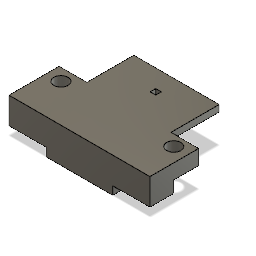
System_Base (Autodesk Fusion 360 archive; units mm, degrees)
design "sensor slit"
Autodesk Fusion 360 part; units mm, degrees
sketch "board contact" plane through (0, 0, 0) normal (0, 1, 0) x (1, 0, 0)
  line L0 (12.7, -1.75) -> (-12.7, -1.75)
  line L1 (-12.7, -1.75) -> (-12.7, 1.75)
  line L2 (-12.7, 1.75) -> (12.7, 1.75)
  line L3 (12.7, 1.75) -> (12.7, -1.75)
  line L4 (61.7395, 0) -> (-97.655, 0) construction
  line L5 (0, -60.5274) -> (0, 48.7233) construction
  line L6 (8.2, 2.75) -> (12.7, 2.75)
  line L7 (12.7, 2.75) -> (12.7, 1.75)
  line L8 (12.7, 1.75) -> (8.2, 1.75)
  line L9 (8.2, 1.75) -> (8.2, 2.75)
  line L10 (-12.7, 3) -> (2.45, 3)
  line L11 (2.45, 3) -> (2.45, 1.75)
  line L12 (2.45, 1.75) -> (-12.7, 1.75)
  line L13 (-12.7, 1.75) -> (-12.7, 3)
  circle A0 centre (10.16, 0.79) radius 1.27
  circle A1 centre (-10.16, 0.79) radius 1.27
  line L14 (-10.16, 0.79) -> (10.16, 0.79) construction
  line L15 (2.45, 9.25) -> (-1.95, 9.25)
  line L16 (-1.95, 9.25) -> (-1.95, 3)
  line L17 (-1.95, 3) -> (2.45, 3)
  line L18 (2.45, 3) -> (2.45, 9.25)
  line L19 (0.5, 7.19) -> (-0.5, 7.19)
  line L20 (-0.5, 7.19) -> (-0.5, 8.19)
  line L21 (-0.5, 8.19) -> (0.5, 8.19)
  line L22 (0.5, 8.19) -> (0.5, 7.19)
  line L23 (7.7, 11.45) -> (-7.7, 11.45)
  line L24 (-7.7, 11.45) -> (-7.7, -1.75)
  line L25 (-7.7, -1.75) -> (7.7, -1.75)
  line L26 (7.7, -1.75) -> (7.7, 11.45)
  line L27 (8.2, 2.75) -> (7.7, 2.75)
  line L28 (-0.5, 7.69) -> (0.5, 7.69) construction
  dimension "d1" = 3.5
  dimension "d2" = 25.4
  dimension "d3" = 4.5
  dimension "d4" = 4.5
  dimension "d7" = 4.75
  dimension "d10" = 20.32
  dimension "d11" = 2.54
  dimension "d12" = 2.54
  dimension "d13" = 10.25
  dimension "d14" = 10.75
  dimension "d15" = 11
  dimension "d17" = 1
  dimension "d18" = 1
  dimension "d20" = 5
  dimension "d21" = 5
  dimension "d22" = 13.2
  dimension "d39" = 9.44
  constraint horizontal L0
  constraint vertical L1
  constraint horizontal L2
  constraint vertical L3
  constraint perpendicular L3 L4
  constraint vertical L5
  constraint coincident origin L5
  constraint coincident origin L4
  constraint symmetric L1 L3 L5
  constraint symmetric L0 L2 L4
  constraint horizontal L6
  constraint vertical L7
  constraint horizontal L8
  constraint vertical L9
  constraint collinear L3 L7
  constraint collinear L2 L8
  constraint horizontal L10
  constraint vertical L11
  constraint horizontal L12
  constraint vertical L13
  constraint collinear L1 L13
  constraint collinear L2 L12
  constraint equal A0 A1
  constraint coincident A1.centre L14.start
  constraint coincident A0.centre L14.end
  constraint horizontal L14
  constraint symmetric L5 A0.centre A1.centre
  constraint horizontal L15
  constraint vertical L16
  constraint horizontal L17
  constraint vertical L18
  constraint collinear L10 L17
  constraint collinear L11 L18
  constraint horizontal L19
  constraint vertical L20
  constraint horizontal L21
  constraint vertical L22
  constraint symmetric L5 L20 L22
  constraint horizontal L23
  constraint vertical L24
  constraint horizontal L25
  constraint vertical L26
  constraint collinear L0 L25
  constraint coincident L26 L27.end
  constraint perpendicular L26 L27
  constraint midpoint L20 L28.start
  constraint midpoint L22 L28.end
  measures "d1" distance of L0.end L1.end
  measures "d2" distance of L0.start L0.end
  measures "d3" distance of L0 L6
  measures "d4" distance of L6.start L6.end
  measures "d7" distance of L0 L10
  measures "d10" distance of A0.centre A1.centre
  measures "d11" distance of L0 A0.centre
  measures "d12" diameter of A0
  measures "d13" distance of L3 L18
  measures "d14" distance of L1 L16
  measures "d15" distance of L0 L15
  measures "d17" distance of L19.start L19.end
  measures "d18" distance of L19.end L20.end
  measures "d20" distance of L3 L26
  measures "d21" distance of L13 L24
  measures "d22" distance of L0 L23
  measures "d39" distance of L0 L28
extrude "Extrude1" add sketch "board contact" along normal blind 3.2 contours L0 L2 L3 L8 A0 L26 | L0 L2 L12 L24 L25 L26 | L2 L6 L7 L8 L9 A0 | L0 L1 L2 L12 A1 L24 | L2 L9 L26 L27 | L2 L10 L11 L15 L16 L18 L23 L24 L26 | L2 L10 L11 L12 L17 L24 | L2 L10 L12 L13 A1 L24 | L10 L15 L16 L17 L18
extrude "Extrude2" cut sketch "board contact" along normal blind 2 contours L2 L9 L26 L27 | L2 L10 L11 L15 L16 L18 L23 L24 L26 | L2 L10 L11 L12 L17 L24 | L10 L15 L16 L17 L18
sketch "vertical extension" plane through (0, 0, 0) normal (0, -1, 0) x (1, 0, 0)
  line L0 (-12.7, -3) -> (-7.7, -3)
  line L1 (-7.7, -1.75) -> (8.2, -1.75)
  line L2 (8.2, -1.75) -> (8.2, -2.75)
  line L3 (8.2, -2.75) -> (12.7, -2.75)
  line L4 (12.7, -2.75) -> (12.7, 1.75)
  line L5 (12.7, 1.75) -> (-12.7, 1.75)
  line L6 (-12.7, 1.75) -> (-12.7, -3)
  circle A0 centre (10.16, -0.79) radius 1.27
  circle A1 centre (-10.16, -0.79) radius 1.27
  line L7 (-6, 6.05) -> (6, 6.05)
  line L8 (6, 6.05) -> (6, 4.55)
  line L9 (6, 4.55) -> (-6, 4.55)
  line L10 (-6, 4.55) -> (-6, 6.05)
  line L11 (0, 1.75) -> (0, -6.45) construction
  line L12 (-12.7, 6.05) -> (12.7, 6.05)
  line L13 (12.7, 6.05) -> (12.7, 1.75)
  line L14 (12.7, 1.75) -> (-12.7, 1.75)
  line L15 (-12.7, 1.75) -> (-12.7, 6.05)
  line L16 (-7.7, -3) -> (-7.7, -1.75)
  dimension "d25" = 12
  dimension "d26" = 1.5
  dimension "d29" = 4.3
  constraint horizontal L7
  constraint vertical L8
  constraint horizontal L9
  constraint vertical L10
  constraint midpoint L5 L11.start
  constraint perpendicular L5 L11
  constraint symmetric L8 L10 L11
  constraint horizontal L12
  constraint vertical L13
  constraint horizontal L14
  constraint vertical L15
  constraint collinear L4 L13
  constraint collinear L6 L15
  constraint collinear L7 L12
  constraint collinear L5 L14
  measures "d25" distance of L7.start L7.end
  measures "d26" distance of L7.end L8.end
  measures "d29" distance of L12.start L5.end
extrude "Extrude4" add sketch "vertical extension" along normal blind -3.2 and the other way blind -1.6 contours L5 L8 L9 L10 L12 L13 L14 L15 | L7 L8 L9 L10 L12
extrude "Extrude3" add sketch "vertical extension" along normal blind 3.1 contours L7 L8 L9 L10 L12
extrude "Extrude6" cut 1 faces at (-2.5667, 0, -0.6331) along direction (0, 1, 0) blind 0.5

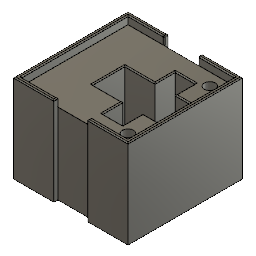
design "button mount v2"
Autodesk Fusion 360 part; units mm, degrees
ref_plane "WorkPlane1" through (0, 0, 12.125) normal (0, 1, 0) x (0, 0, 1)
sketch "face" plane through (0, 0, 12.125) normal (0, 1, 0) x (0, 0, 1)
  line L0 (0, 23) -> (0, -23) construction
  line L1 (-28, 0) -> (21, 0) construction
  line L2 (0, 13.2) -> (-13.2, 13.2)
  line L3 (9, 2.7) -> (4, 2.7)
  line L4 (0, -14.2) -> (0, -13.2)
  line L5 (14.2, -14.2) -> (13.2, -14.2)
  line L6 (13.2, -4.2) -> (14.2, -4.2)
  line L7 (13.2, 13.2) -> (13.2, -13.2)
  line L8 (4, 7.7) -> (4, 13.2)
  line L9 (13.2, -13.2) -> (13.2, -4.2)
  line L10 (-13.2, -13.2) -> (-13.2, -4.2)
  line L11 (0, -13.2) -> (13.2, -13.2)
  line L12 (14.2, -4.2) -> (14.2, -14.2)
  line L13 (12.7, 12.7) -> (12.7, -12.7) construction
  line L14 (9, 7.7) -> (9, 2.7)
  line L15 (-4, 2.7) -> (-4, -4.8)
  line L16 (4, 7.7) -> (9, 7.7)
  line L17 (0, 14.2) -> (0, 13.2)
  line L18 (0, 13.2) -> (13.2, 13.2)
  circle A0 centre (10.16, 10.16) radius 1.375
  line L19 (4, -4.8) -> (4, 2.7)
  line L20 (-13.2, 13.2) -> (13.2, 13.2)
  line L21 (-12.7, -12.7) -> (-12.7, 12.7) construction
  line L22 (-13.2, 13.2) -> (-13.2, 4.2)
  line L23 (14.2, 14.2) -> (13.2, 14.2)
  line L24 (13.2, -13.2) -> (-13.2, -13.2)
  line L25 (13.2, 14.2) -> (0, 14.2)
  line L26 (-9, 2.7) -> (-9, 7.7)
  line L27 (-4, 2.7) -> (-9, 2.7)
  line L28 (13.2, 13.2) -> (13.2, 4.2)
  line L29 (4, 13.2) -> (-4, 13.2)
  line L30 (13.2, -14.2) -> (0, -14.2)
  line L31 (13.2, 4.2) -> (14.2, 4.2)
  line L32 (14.2, 4.2) -> (14.2, 14.2)
  line L33 (-9, 7.7) -> (-4, 7.7)
  line L34 (-14.2, -14.2) -> (-13.2, -14.2)
  line L35 (12.7, -12.7) -> (-12.7, -12.7) construction
  line L36 (-13.2, 4.2) -> (-14.2, 4.2)
  line L37 (-12.7, 0) -> (12.7, 0) construction
  line L38 (-13.2, -14.2) -> (0, -14.2)
  line L39 (-4, -4.8) -> (4, -4.8)
  line L40 (0, -14.2) -> (0, -13.2)
  line L41 (-13.2, -4.2) -> (-14.2, -4.2)
  line L42 (0, 12.7) -> (0, -12.7) construction
  line L43 (0, 14.2) -> (0, 13.2)
  line L44 (-14.2, -4.2) -> (-14.2, -14.2)
  line L45 (-12.7, 12.7) -> (12.7, 12.7) construction
  line L46 (-14.2, 14.2) -> (-13.2, 14.2)
  line L47 (-14.2, 4.2) -> (-14.2, 14.2)
  line L48 (0, -13.2) -> (-13.2, -13.2)
  line L49 (-13.2, 14.2) -> (0, 14.2)
  circle A1 centre (-10.16, 10.16) radius 1.375
  line L50 (-13.2, -13.2) -> (-13.2, 13.2)
  line L51 (-4, 13.2) -> (-4, 7.7)
  circle A2 centre (0, 5.25) radius 4.5 construction
  dimension "d284" = 25.4
  dimension "d285" = 25.4
  dimension "d286" = 2.75
  dimension "d287" = 2.54
  dimension "d288" = 2.54
  dimension "d289" = 2.54
  dimension "d290" = 2.54
  dimension "d291" = 26.4
  dimension "d292" = 26.4
  dimension "d293" = 18
  dimension "d294" = 8
  dimension "d295" = 5
  dimension "d296" = 10.5
  dimension "d297" = 18
  dimension "d298" = 10
  dimension "d299" = 14.2
  dimension "d300" = 1
  dimension "d301" = 1
  dimension "d31" = 17.95
  dimension "d32" = 9
  constraint vertical L0
  constraint horizontal L1
  constraint coincident origin L1
  constraint coincident origin L0
  constraint horizontal L45
  constraint vertical L13
  constraint horizontal L35
  constraint vertical L21
  constraint equal A0 A1
  constraint horizontal L20
  constraint vertical L7
  constraint horizontal L24
  constraint vertical L50
  constraint midpoint L42.start L45
  constraint midpoint L42.end L35
  constraint midpoint L37.start L21
  constraint midpoint L37.end L13
  constraint symmetric L7 L42 L50
  constraint symmetric L20 L24 L37
  constraint horizontal L39
  constraint vertical L19
  constraint horizontal L29
  constraint vertical L51
  constraint collinear L20 L29
  constraint horizontal L33
  constraint vertical L14
  constraint horizontal L3
  constraint vertical L26
  constraint coincident L15.start L3
  constraint collinear L15 L51
  constraint collinear L16 L33
  constraint collinear L3 L27
  constraint collinear L8 L19
  constraint horizontal L46
  constraint vertical L22
  constraint horizontal L36
  constraint vertical L47
  constraint horizontal L49
  constraint vertical L43
  constraint horizontal L2
  constraint collinear L2 L20
  constraint collinear L22 L50
  constraint symmetric L46.start L23.start L42
  constraint symmetric L46.end L23.end L42
  constraint symmetric L28.end L22.end L42
  constraint symmetric L31.end L36.end L42
  constraint symmetric L17.start L25.end L42
  constraint symmetric L2.start L17.end L42
  constraint symmetric L2.end L7.start L42
  constraint symmetric L34.start L46.start L37
  constraint symmetric L34.end L46.end L37
  constraint symmetric L10.end L22.end L37
  constraint symmetric L36.end L41.end L37
  constraint symmetric L17.start L4.start L37
  constraint symmetric L2.start L4.end L37
  constraint symmetric L10.start L2.end L37
  constraint symmetric L28.end L6.start L37
  constraint symmetric L31.end L6.end L37
  constraint symmetric L23.start L5.start L37
  constraint symmetric L23.end L5.end L37
  constraint symmetric L7.start L7.end L37
  constraint collinear L0 L42
  constraint collinear L1 L37
  constraint coincident L42 A2.centre
  measures "d284" distance of L13.start L21.end
  measures "d285" distance of L13.start L13.end
  measures "d286" diameter of A1
  measures "d287" distance of A1.centre L45
  measures "d288" distance of A1.centre L21
  measures "d289" distance of A0.centre L45
  measures "d290" distance of A0.centre L13
  measures "d291" distance of L7.start L2.end
  measures "d292" distance of L7.end L7.start
  measures "d293" distance of L19.start L8.end
  measures "d294" distance of L19.start L15.end
  measures "d295" distance of L14.start L3.start
  measures "d296" distance of L3 L20
  measures "d297" distance of L3.start L26.start
  measures "d298" distance of L46.start L36.end
  measures "d299" distance of L43 L47
  measures "d300" distance of L17.start L2.start
  measures "d301" distance of L36.end L22.end
  measures "d31" distance of L35 A2.centre
  measures "d32" diameter of A2
ref_plane "WorkPlane2" through (0, -20, 0) normal (0, 1, 0) x (0, 0, 1)
extrude "Extrude1" add sketch "face" against normal up to surface (20 mm away) contours L2 L3 L7 L8 L9 L10 L11 L14 L15 L16 L18 L19 L20 L22 L24 L26 L27 L28 L33 L39 L48 L50 L51 | A0 | A1
extrude "Extrude3" cut sketch "face" against normal blind 13 contours A0 | A1
extrude "Extrude4" add sketch "face" along normal blind 2 and the other way up to surface (20 mm away) contours L2 L17 L20 L22 L29 L36 L43 L46 L47 L49 L50 | L7 L17 L18 L20 L23 L25 L28 L29 L31 L32 L43 | L4 L10 L24 L34 L38 L40 L41 L44 L48 L50 | L4 L5 L6 L7 L9 L11 L12 L24 L30 L40
fillet "Fillet3" radius 0.25 8 edges at (8.7, 2, -1.075) (4.2, 1, -1.075) (-4.2, 1, -1.075) (-8.7, 2, -1.075) (-13.2, 2, 12.125) (13.2, 2, 12.125) (-8.7, 2, 25.325) (8.7, 2, 25.325)
fillet "Fillet3" radius 0.25 11 edges at (10.45, 0, 8.125) (7.7, 0, 5.625) (5.2, 0, 3.125) (2.7, 0, 5.625) (-1.05, 0, 8.125) (-4.8, 0, 12.125) (-1.05, 0, 16.125) (2.7, 0, 18.625) (5.2, 0, 21.125) (7.7, 0, 18.625) (10.45, 0, 16.125)
fillet "Fillet3" radius 0.25 10 edges at (9.2, 2, -2.075) (4.2, 2, -1.575) (-4.2, 2, -1.575) (-9.2, 2, -2.075) (-14.2, 2, 12.125) (-9.2, 2, 26.325) (-4.2, 2, 25.825) (4.2, 2, 25.825) (9.2, 2, 26.325) (14.2, 2, 12.125)
equation "FACE_DEG = 0 deg"
equation "d289 = d263"
equation "d290 = d264"
equation "d291 = 26.10 mm + 2 * 0.15 mm"
equation "d292 = 26.10 mm + 2 * 0.15 mm"
equation "HEIGHT = -20 mm"

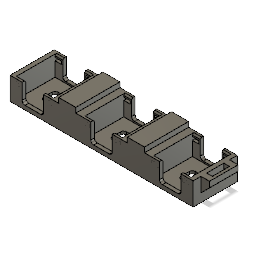
design "magnet storage v4"
Autodesk Fusion 360 part; units mm, degrees
sketch "base" plane through (0, 0, 0) normal (0, 1, 0) x (1, 0, 0)
  line L0 (-64, 15.5) -> (64, 15.5)
  line L1 (64, 15.5) -> (64, -15.5)
  line L2 (64, -15.5) -> (-64, -15.5)
  line L3 (-64, -15.5) -> (-64, 15.5)
  line L4 (64, 0) -> (-64, 0) construction
  line L5 (0, 15.5) -> (0, -15.5) construction
  line L6 (-61, 13) -> (-35, 13)
  line L7 (-35, 13) -> (-35, -13)
  line L8 (-35, -13) -> (-61, -13)
  line L9 (-61, -13) -> (-61, 13)
  line L10 (-53, 5) -> (-43, 5)
  line L11 (-43, 5) -> (-43, -5)
  line L12 (-43, -5) -> (-53, -5)
  line L13 (-53, -5) -> (-53, 5)
  line L14 (-48, 13) -> (-48, -13) construction
  line L15 (-13, 13) -> (13, 13)
  line L16 (-13, -13) -> (-13, 13)
  line L17 (13, -13) -> (-13, -13)
  line L18 (5, -5) -> (-5, -5)
  line L19 (-5, -5) -> (-5, 5)
  line L20 (-5, 5) -> (5, 5)
  line L21 (5, 5) -> (5, -5)
  line L22 (13, 13) -> (13, -13)
  line L23 (35, 13) -> (61, 13)
  line L24 (35, -13) -> (35, 13)
  line L25 (61, -13) -> (35, -13)
  line L26 (53, -5) -> (43, -5)
  line L27 (43, -5) -> (43, 5)
  line L28 (43, 5) -> (53, 5)
  line L29 (53, 5) -> (53, -5)
  line L30 (61, 13) -> (61, -13)
  dimension "d2" = 31
  dimension "d3" = 26
  dimension "d4" = 10
  dimension "d5" = 3
  dimension "d8" = 48
  dimension "d9" = 0
  dimension "d86" = 3
  constraint horizontal L0
  constraint vertical L1
  constraint horizontal L2
  constraint vertical L3
  constraint midpoint L1 L4.start
  constraint midpoint L3 L4.end
  constraint midpoint L0 L5.start
  constraint midpoint L2 L5.end
  constraint coincident origin L5
  constraint coincident origin L4
  constraint horizontal L6
  constraint vertical L7
  constraint horizontal L8
  constraint vertical L9
  constraint horizontal L10
  constraint vertical L11
  constraint horizontal L12
  constraint vertical L13
  constraint equal L6 L7
  constraint equal L10 L11
  constraint symmetric L4 L6 L8
  constraint midpoint L6 L14.start
  constraint midpoint L8 L14.end
  constraint symmetric L4 L10 L12
  constraint symmetric L11 L13 L14
  measures "d2" distance of L0.start L2.end
  measures "d3" distance of L6.start L8.end
  measures "d4" distance of L10.start L10.end
  measures "d5" distance of L3 L9
  measures "d86" distance of L1 L30
extrude "Extrude1" add sketch "base" along normal blind 2 contours L6 L7 L8 L9 | L15 L16 L17 L22 | L23 L24 L25 L30 makes body 1 at (10.3333, 0, -1.6667) makes body 2 at (58.3333, 0, 1.6667) makes body 3 at (-58.3333, 0, 1.6667)
extrude "Extrude2" add sketch "base" along normal blind 12 contours L0 L1 L2 L3 bodies 1 2 3
sketch "access slots" plane through (0, 0, 15.5) normal (0, 0, 1) x (1, 0, 0)
  line L0 (-64, 0) -> (64, 0)
  line L1 (64, 0) -> (64, 12)
  line L2 (64, 12) -> (-64, 12)
  line L3 (-64, 12) -> (-64, 0)
  line L4 (-42.5, 3) -> (-53.5, 3)
  line L5 (-55.5, 5) -> (-55.5, 12)
  line L6 (-55.5, 12) -> (-40.5, 12)
  line L7 (-40.5, 12) -> (-40.5, 5)
  line L8 (64, 0) -> (-64, 0)
  line L9 (-48, 12) -> (-48, 3) construction
  arc A0 (-55.5, 5) -> (-53.5, 3) centre (-53.5, 5) ccw
  arc A1 (-42.5, 3) -> (-40.5, 5) centre (-42.5, 5) ccw
  line L10 (-7.5, 5) -> (-7.5, 12)
  line L11 (-7.5, 12) -> (7.5, 12)
  arc A2 (-7.5, 5) -> (-5.5, 3) centre (-5.5, 5) ccw
  line L12 (5.5, 3) -> (-5.5, 3)
  arc A3 (5.5, 3) -> (7.5, 5) centre (5.5, 5) ccw
  line L13 (7.5, 12) -> (7.5, 5)
  line L14 (40.5, 5) -> (40.5, 12)
  line L15 (40.5, 12) -> (55.5, 12)
  arc A4 (40.5, 5) -> (42.5, 3) centre (42.5, 5) ccw
  line L16 (53.5, 3) -> (42.5, 3)
  arc A5 (53.5, 3) -> (55.5, 5) centre (53.5, 5) ccw
  line L17 (55.5, 12) -> (55.5, 5)
  point P0 (-61, 12)
  point P1 (-13, 12)
  point P2 (35, 12)
  point P3 (35, 15)
  dimension "d20" = 3
  dimension "d21" = 15
  dimension "d22" = 13
  dimension "d23" = 2
  dimension "d26" = 48
  dimension "d27" = 0
  constraint horizontal L4
  constraint vertical L5
  constraint horizontal L6
  constraint vertical L7
  constraint midpoint L6 L9.start
  constraint collinear L2 L6
  constraint coincident L4 L9.end
  constraint tangent L4 A0
  constraint tangent L5 A0
  constraint tangent L4 A1
  constraint tangent L7 A1
  constraint equal A0 A1
  constraint midpoint L4 L9.end
  measures "d20" distance of L4 L8
  measures "d21" distance of L5.end L6.end
  measures "d22" distance of P0 L9
  measures "d23" radius of A0
extrude "Extrude3" cut sketch "access slots" against normal up to surface (31 mm away) contours L2 L4 L5 L6 L7 A0 A1 | L2 L14 L15 A4 L16 A5 L17 | L2 L10 L11 A2 L12 A3 L13 bodies 1
fillet "Fillet1" radius 2 12 edges at (-43, 1, 5) (-53, 1, 5) (-53, 1, -5) (-43, 1, -5) (5, 1, -5) (5, 1, 5) (-5, 1, 5) (-5, 1, -5) (43, 1, -5) (43, 1, 5) (53, 1, -5) (53, 1, 5) on bodies 1
ref_plane "WorkPlane1" through (0, 12, 0) normal (0, 1, 0) x (0, 0, 1)
sketch "cover indents" plane through (-24, 12, 0) normal (0, 1, 0) x (1, 0, 0)
  circle A0 centre (-5, 9.5) radius 1.4
  circle A1 centre (-5, 9.5) radius 3
  line L0 (16.5, 15.5) -> (-16.5, 15.5)
  line L1 (-5, 12.5) -> (-11, 12.5)
  line L2 (11, -13) -> (-11, -13)
  circle A2 centre (5, 9.5) radius 1.4
  circle A3 centre (5, 9.5) radius 3
  line L3 (-5, 9.5) -> (5, 9.5) construction
  line L4 (5, 12.5) -> (11, 12.5)
  line L5 (-11, 13) -> (-11, -13)
  line L6 (11, -13) -> (11, 13)
  line L7 (-11, -13) -> (-16.5, -13)
  line L8 (-2, 9.5) -> (-2, 8)
  line L9 (2, 9.5) -> (2, 8)
  circle A4 centre (43, -9.5) radius 1.4
  circle A5 centre (43, -9.5) radius 3
  line L10 (37, 13) -> (37, -13)
  line L11 (31.5, -15.5) -> (64.5, -15.5)
  circle A6 centre (53, -9.5) radius 1.4
  circle A7 centre (53, -9.5) radius 3
  line L12 (43, -9.5) -> (53, -9.5) construction
  line L13 (59, -13) -> (59, 13) construction
  line L14 (43, -12.5) -> (37, -12.5)
  line L15 (59, -12.5) -> (53, -12.5)
  line L16 (37, 13) -> (59, 13)
  line L17 (37, 13) -> (37, -12.5)
  line L18 (59, -13) -> (59, 13)
  line L19 (46, -9.5) -> (46, -6.5)
  line L20 (46, -6.5) -> (50, -6.5)
  line L21 (50, -6.5) -> (50, -9.5)
  line L22 (-2, 8) -> (2, 8)
  dimension "d33" = 2.8
  dimension "d34" = 6
  dimension "d35" = 6
  dimension "d37" = 6
  dimension "d38" = 6
  dimension "d57" = 6
  dimension "d58" = 6
  dimension "d59" = 6
  dimension "d84" = 1.5
  constraint concentric A0 A1
  constraint coincident A1 L1.start
  constraint horizontal L1
  constraint equal A0 A2
  constraint concentric A2 A3
  constraint equal A1 A3
  constraint coincident A0.centre A1.centre
  constraint coincident A2.centre A3.centre
  constraint horizontal L3
  constraint coincident A3 L4.start
  constraint horizontal L4
  constraint coincident L4.end L6
  constraint coincident L1.end L5
  constraint tangent A1 L1
  constraint tangent A3 L4
  constraint coincident L2.end L5
  constraint coincident L2.start L6
  constraint collinear L2 L7
  constraint coincident A1 L8.start
  constraint coincident L3 L8.start
  constraint tangent A1 L8
  constraint coincident A3 L9.start
  constraint coincident L3 L9.start
  constraint tangent A3 L9
  constraint equal A2 A4
  constraint concentric A4 A5
  constraint equal A3 A5
  constraint concentric A6 A7
  constraint equal A4 A6
  constraint equal A5 A7
  constraint coincident A4.centre A5.centre
  constraint coincident A6.centre A7.centre
  constraint horizontal L12
  constraint coincident A5 L14.start
  constraint coincident L10 L14.end
  constraint tangent A5 L14
  constraint horizontal L14
  constraint coincident L13 L15.start
  constraint coincident A7 L15.end
  constraint perpendicular L13 L15
  constraint tangent A7 L15
  constraint coincident L10.start L16.start
  constraint coincident L13.end L16.end
  constraint coincident L13.start L18.start
  constraint coincident A5 L19.start
  constraint coincident L12 L19.start
  constraint tangent A5 L19
  constraint perpendicular L18 L20
  constraint coincident A7 L21.end
  constraint coincident L12 L21.end
  constraint tangent A7 L21
  constraint tangent A5 L20
  constraint equal L8 L9
  measures "d33" diameter of A0
  measures "d34" diameter of A1
  measures "d35" distance of A0.centre L0
  measures "d37" distance of A0.centre L5
  measures "d38" distance of A2.centre L6
  measures "d57" distance of A4.centre L10
  measures "d58" distance of A4.centre L11
  measures "d59" distance of A6.centre L13
  measures "d84" distance of L9.start L9.end
extrude "Extrude9" add 2 faces at (-63, 12, -4.3333) (63, 12, 4.3333) along direction (0, 1, 0) blind 4 on bodies 1 bodies 1
sketch "left top" plane through (0, 12, 0) normal (0, 1, 0) x (-1, 0, 0)
  line L0 (-7.5, -15.5) -> (-7.5, -13)
  line L1 (-7.5, -13) -> (-13, -13)
  line L2 (-13, -13) -> (-13, 13)
  line L3 (-13, 13) -> (-7.5, 13)
  line L4 (-7.5, 13) -> (-7.5, 15.5)
  line L5 (-7.5, 15.5) -> (-40.5, 15.5)
  line L6 (-40.5, 15.5) -> (-40.5, 13)
  line L7 (-40.5, 13) -> (-35, 13)
  line L8 (-35, 13) -> (-35, -13)
  line L9 (-35, -13) -> (-40.5, -13)
  line L10 (-40.5, -13) -> (-40.5, -15.5)
  line L11 (-40.5, -15.5) -> (-7.5, -15.5)
  line L12 (-30, 15.5) -> (-30, -15.5)
  line L13 (-18, 15.5) -> (-18, -15.5)
  dimension "d94" = 5
  dimension "d95" = 5
  dimension "d138" = 12
  constraint coincident L5 L12.start
  constraint coincident L11 L12.end
  constraint perpendicular L11 L12
  constraint coincident L5 L13.start
  constraint coincident L11 L13.end
  constraint perpendicular L11 L13
  measures "d94" distance of L8 L12
  measures "d95" distance of L2 L13
  measures "d138" distance of L12 L13
extrude "Extrude11" add sketch "left top" along normal blind 4 contours L5 L6 L7 L8 L9 L10 L11 L12 bodies 1
ref_plane "WorkPlane4" through (48, 9, 13) normal (0, 0, -1) x (-1, 0, 0)
sketch "left prong holes" plane through (37.75, 13.75, 13) normal (0, 0, -1) x (1, 0, 0)
  line L0 (1.75, -0.25) -> (-2.75, -0.25)
  line L1 (-2.75, -0.25) -> (-2.75, 2)
  line L2 (-2.75, 2) -> (1.75, 2)
  line L3 (1.75, 2) -> (1.75, -0.25)
  line L4 (2.75, -2.25) -> (2.75, 8.75)
  line L5 (18.75, -0.25) -> (23.25, -0.25)
  line L6 (23.25, -0.25) -> (23.25, 2)
  line L7 (23.25, 2) -> (18.75, 2)
  line L8 (18.75, 2) -> (18.75, -0.25)
  line L9 (17.75, 8.75) -> (17.75, -2.25)
  line L10 (-7.75, -2.25) -> (2.75, -2.25)
  line L11 (17.75, -2.25) -> (26.25, -2.25)
  dimension "d119" = 1
  dimension "d120" = 4.5
  dimension "d121" = 2.25
  dimension "d123" = 1
  dimension "d125" = 2.25
  dimension "d132" = 2
  dimension "d133" = 2
  constraint horizontal L0
  constraint vertical L1
  constraint horizontal L2
  constraint vertical L3
  constraint horizontal L5
  constraint vertical L6
  constraint horizontal L7
  constraint vertical L8
  constraint equal L0 L5
  measures "d119" distance of L3 L4
  measures "d120" distance of L0.start L0.end
  measures "d121" distance of L0.end L1.end
  measures "d123" distance of L8 L9
  measures "d125" distance of L5.start L7.end
  measures "d132" distance of L0 L10
  measures "d133" distance of L5 L11
extrude "Extrude16" cut sketch "left prong holes" against normal blind 2 bodies 1
mirror "Mirror1" about plane through (0, 0, 0) normal (0, 0, 1) of "Extrude16"
sketch "right top" plane through (0, 12, 0) normal (0, 1, 0) x (-1, 0, 0)
  line L0 (40.5, -15.5) -> (40.5, -13)
  line L1 (40.5, -13) -> (35, -13)
  line L2 (35, -13) -> (35, 13)
  line L3 (35, 13) -> (40.5, 13)
  line L4 (40.5, 13) -> (40.5, 15.5)
  line L5 (40.5, 15.5) -> (7.5, 15.5)
  line L6 (7.5, 15.5) -> (7.5, 13)
  line L7 (7.5, 13) -> (13, 13)
  line L8 (13, 13) -> (13, -13)
  line L9 (13, -13) -> (7.5, -13)
  line L10 (7.5, -13) -> (7.5, -15.5)
  line L11 (7.5, -15.5) -> (40.5, -15.5)
  line L12 (18, 15.5) -> (18, -15.5)
  line L13 (30, 15.5) -> (30, -15.5)
  dimension "d141" = 5
  dimension "d142" = 5
  constraint coincident L5 L12.start
  constraint coincident L11 L12.end
  constraint perpendicular L11 L12
  constraint coincident L5 L13.start
  constraint coincident L11 L13.end
  constraint perpendicular L11 L13
  measures "d141" distance of L8 L12
  measures "d142" distance of L2 L13
extrude "Extrude17" add sketch "right top" sketch "left top" along normal blind 7.5 contours L5 L11 L12 L13 of sketch 2 contours L5 L11 L12 L13 bodies 1
extrude "Extrude18" add sketch "left top" 2 faces at (-16.3333, 12, -4.3333) (-31.6667, 12, 4.3333) along normal blind 4 contours L0 L1 L2 L3 L4 L5 L11 L13 on bodies 1 bodies 1
sketch "middle prong holes" plane through (0, 0, 13) normal (0, 0, -1) x (-1, 0, 0)
  line L0 (-7.5, 5) -> (-7.5, 16)
  line L1 (-7.5, 16) -> (-13, 16)
  line L2 (-13, 16) -> (-13, 2)
  line L3 (-13, 2) -> (13, 2)
  line L4 (13, 2) -> (13, 16)
  line L5 (13, 16) -> (7.5, 16)
  line L6 (7.5, 16) -> (7.5, 5)
  arc A0 (5.5, 3) -> (7.5, 5) centre (5.5, 5) ccw
  line L7 (5.5, 3) -> (-5.5, 3)
  arc A1 (-7.5, 5) -> (-5.5, 3) centre (-5.5, 5) ccw
  line L8 (-13, 14) -> (-8.5, 14)
  line L9 (-8.5, 14) -> (-8.5, 12)
  line L10 (-8.5, 12) -> (-13, 12)
  line L11 (-13, 12) -> (-13, 14)
  line L12 (8.5, 14) -> (13, 14)
  line L13 (13, 14) -> (13, 12)
  line L14 (13, 12) -> (8.5, 12)
  line L15 (8.5, 12) -> (8.5, 14)
  dimension "d145" = 2
  dimension "d146" = 1
  dimension "d147" = 4.5
  dimension "d148" = 2
  dimension "d149" = 1
  constraint horizontal L8
  constraint vertical L9
  constraint horizontal L10
  constraint vertical L11
  constraint horizontal L12
  constraint vertical L13
  constraint horizontal L14
  constraint vertical L15
  constraint collinear L8 L12
  constraint collinear L10 L14
  constraint equal L8 L12
  measures "d145" distance of L1 L8
  measures "d146" distance of L0 L9
  measures "d147" distance of L8.start L8.end
  measures "d148" distance of L8.end L9.end
  measures "d149" distance of L6 L15
sketch "right prong holes" plane through (0, 0, 13) normal (0, 0, -1) x (-1, 0, 0)
  line L0 (40.5, 5) -> (40.5, 16)
  line L1 (40.5, 16) -> (35, 16)
  line L2 (35, 16) -> (35, 2)
  line L3 (35, 2) -> (61, 2)
  line L4 (61, 2) -> (61, 16)
  line L5 (61, 16) -> (55.5, 16)
  line L6 (55.5, 16) -> (55.5, 5)
  arc A0 (53.5, 3) -> (55.5, 5) centre (53.5, 5) ccw
  line L7 (53.5, 3) -> (42.5, 3)
  arc A1 (40.5, 5) -> (42.5, 3) centre (42.5, 5) ccw
  line L8 (35, 14) -> (39.5, 14)
  line L9 (39.5, 14) -> (39.5, 12)
  line L10 (39.5, 12) -> (35, 12)
  line L11 (35, 12) -> (35, 14)
  line L12 (56.5, 14) -> (61, 14)
  line L13 (61, 14) -> (61, 12)
  line L14 (61, 12) -> (56.5, 12)
  line L15 (56.5, 12) -> (56.5, 14)
  dimension "d150" = 1
  dimension "d151" = 2
  dimension "d152" = 4.5
  dimension "d153" = 2
  dimension "d154" = 1
  constraint horizontal L8
  constraint vertical L9
  constraint horizontal L10
  constraint vertical L11
  constraint horizontal L12
  constraint vertical L13
  constraint horizontal L14
  constraint vertical L15
  constraint equal L8 L12
  constraint collinear L8 L12
  constraint collinear L10 L14
  measures "d150" distance of L0 L9
  measures "d151" distance of L1 L8
  measures "d152" distance of L8.start L8.end
  measures "d153" distance of L8.end L9.end
  measures "d154" distance of L6 L15
extrude "Extrude19" cut sketch "middle prong holes" sketch "right prong holes" along normal blind 28 and the other way blind 2 contours L2 L8 L9 L10 L11 | L4 L12 L13 L14 L15 of sketch 2 contours L2 L8 L9 L10 L11 | L4 L12 L13 L14 L15 bodies 1
chamfer "Chamfer2" distance 1 angle 45 2 edges at (37.75, 16, 13) (58.25, 16, 13) on bodies 1
chamfer "Chamfer2" distance 1 angle 45 2 edges at (37.75, 16, -13) (58.25, 16, -13) on bodies 1
chamfer "Chamfer2" distance 1 angle 45 8 edges at (10.25, 16, 13) (-10.25, 16, 13) (10.25, 16, -13) (-10.25, 16, -13) (-37.75, 16, 13) (-58.25, 16, 13) (-58.25, 16, -13) (-37.75, 16, -13) on bodies 1
sketch "handle" plane through (64, 0, 0) normal (1, 0, 0) x (0, 0, -1)
  line L0 (-15.5, 0) -> (15.5, 0)
  line L1 (15.5, 0) -> (15.5, 16)
  line L2 (-15.5, 16) -> (-15.5, 0)
  line L3 (-10, 16) -> (10, 16)
  line L4 (10, 16) -> (10, 12)
  line L5 (10, 12) -> (-10, 12)
  line L6 (-10, 12) -> (-10, 16)
  line L7 (0, 19) -> (0, 0) construction
  line L8 (-6, 16) -> (-6, 12)
  line L9 (6, 16) -> (6, 12)
  line L10 (15.5, 16) -> (-15.5, 16)
  dimension "d73" = 20
  dimension "d74" = 4
  dimension "d76" = 4
  dimension "d77" = 4
  constraint horizontal L3
  constraint vertical L4
  constraint horizontal L5
  constraint vertical L6
  constraint coincident L7.end origin
  constraint symmetric L4 L6 L7
  constraint coincident L3 L8.start
  constraint coincident L5 L8.end
  constraint perpendicular L5 L8
  constraint coincident L3 L9.start
  constraint coincident L5 L9.end
  constraint perpendicular L5 L9
  measures "d73" distance of L3.start L3.end
  measures "d74" distance of L3.start L5.end
  measures "d76" distance of L4 L9
  measures "d77" distance of L6 L8
extrude "Extrude7" add sketch "handle" along normal blind 6 contours L3 L5 L6 L8 L10 | L3 L4 L5 L9 L10 | L3 L5 L8 L9 L10 bodies 1
extrude "Extrude8" cut sketch "handle" along normal blind 4 contours L3 L5 L8 L9 L10 bodies 1
draft "Draft1" angle 45 neutral plane through (70, 0, 0) pull (1, 0, 0) 1 faces at (67.3333, 12, -8.6667) on bodies 1
equation "d38 = d37"
equation "d57 = d37"
equation "d58 = d35"
equation "d59 = d37"
equation "d77 = d76"
equation "d95 = d94"
equation "d123 = d119"
equation "d142 = d141"
equation "d149 = d146"
equation "d154 = d150"

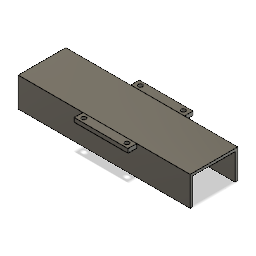
design "magnet storage cover"
Autodesk Fusion 360 part; units mm, degrees
sketch "base" plane through (0, 0, 0) normal (0, 1, 0) x (1, 0, 0)
  line L0 (-67, 15.5) -> (67, 15.5) construction
  line L1 (67, 15.5) -> (67, -15.5) construction
  line L2 (67, -15.5) -> (-67, -15.5) construction
  line L3 (-67, -15.5) -> (-67, 15.5) construction
  line L4 (0, 15.5) -> (0, -15.5) construction
  line L5 (-67, 0) -> (67, 0) construction
  line L6 (-69.25, 17.75) -> (58.75, 17.75)
  line L7 (58.75, 17.75) -> (58.75, 15.75)
  line L8 (58.75, 15.75) -> (-69.25, 15.75)
  line L9 (-69.25, 15.75) -> (-69.25, 17.75)
  line L10 (-69.25, -15.75) -> (58.75, -15.75)
  line L11 (58.75, -15.75) -> (58.75, -17.75)
  line L12 (58.75, -17.75) -> (-69.25, -17.75)
  line L13 (-69.25, -17.75) -> (-69.25, -15.75)
  line L14 (-69.25, 15.75) -> (-69.25, -15.75)
  line L15 (-67.25, -15.75) -> (-67.25, 15.75)
  dimension "d1" = 134
  dimension "d2" = 31
  dimension "d3" = 128
  dimension "d4" = 2
  dimension "d5" = 2
  dimension "margin" = 0.25
  dimension "d7" = 0.25
  dimension "d8" = 0.25
  constraint horizontal L0
  constraint vertical L1
  constraint horizontal L2
  constraint vertical L3
  constraint midpoint L0 L4.start
  constraint midpoint L2 L4.end
  constraint midpoint L3 L5.start
  constraint midpoint L1 L5.end
  constraint coincident origin L5
  constraint coincident origin L4
  constraint horizontal L6
  constraint vertical L7
  constraint horizontal L8
  constraint vertical L9
  constraint horizontal L10
  constraint vertical L11
  constraint horizontal L12
  constraint vertical L13
  constraint collinear L7 L11
  constraint collinear L9 L13
  constraint coincident L10 L15.start
  constraint coincident L8 L15.end
  constraint perpendicular L8 L15
  constraint equal L9 L13
  measures "d1" distance of L0.start L0.end
  measures "d2" distance of L0.start L2.end
  measures "d3" distance of L6.start L6.end
  measures "d4" distance of L6.start L8.end
  measures "d5" distance of L14 L15
  measures "margin" distance of L3 L15
  measures "d7" distance of L2 L10
  measures "d8" distance of L0 L8
extrude "Extrude1" add sketch "base" along normal blind 20 makes body 1
sketch "top" plane through (0, 20, 0) normal (0, 1, 0) x (-1, 0, 0)
  line L0 (-58.75, 15.75) -> (67.25, 15.75)
  line L1 (67.25, 15.75) -> (67.25, -15.75)
  line L2 (67.25, -15.75) -> (-58.75, -15.75)
  line L3 (-58.75, -15.75) -> (-58.75, -17.75)
  line L4 (-58.75, -17.75) -> (69.25, -17.75)
  line L5 (69.25, -17.75) -> (69.25, 17.75)
  line L6 (69.25, 17.75) -> (-58.75, 17.75)
  line L7 (-58.75, 17.75) -> (-58.75, 15.75)
  line L8 (69.25, -17.75) -> (-58.75, -17.75)
  line L9 (-58.75, -17.75) -> (-58.75, 17.75)
  line L10 (-58.75, 17.75) -> (69.25, 17.75)
  line L11 (69.25, 17.75) -> (69.25, -17.75)
  constraint horizontal L8
  constraint vertical L9
  constraint horizontal L10
  constraint vertical L11
  constraint collinear L3 L9
  constraint collinear L5 L11
  constraint collinear L4 L8
  constraint collinear L6 L10
extrude "Extrude2" add sketch "top" along normal blind 2 bodies 1
sketch "wing supports" plane through (0, 22, 0) normal (0, 1, 0) x (-1, 0, 0)
  line L0 (69.25, 17.75) -> (-58.75, 17.75)
  line L1 (-58.75, 17.75) -> (-58.75, -17.75)
  line L2 (-58.75, -17.75) -> (69.25, -17.75)
  line L3 (69.25, -17.75) -> (69.25, 17.75)
  line L4 (21, -24.25) -> (-19, -24.25)
  line L5 (-19, -24.25) -> (-19, -17.75)
  line L6 (-19, -17.75) -> (21, -17.75)
  line L7 (21, -17.75) -> (21, -24.25)
  line L8 (21, 17.75) -> (-19, 17.75)
  line L9 (-19, 17.75) -> (-19, 24.25)
  line L10 (-19, 24.25) -> (21, 24.25)
  line L11 (21, 24.25) -> (21, 17.75)
  circle A0 centre (17, 21) radius 1.55
  circle A1 centre (-15, 21) radius 1.55
  line L12 (17, 21) -> (-15, 21) construction
  circle A2 centre (17, -21) radius 1.55
  circle A3 centre (-15, -21) radius 1.55
  line L13 (17, -21) -> (-15, -21) construction
  circle A4 centre (17, 21) radius 2.75
  circle A5 centre (-15, 21) radius 2.75
  circle A6 centre (17, -21) radius 2.75
  circle A7 centre (-15, -21) radius 2.75
  dimension "d13" = 6.5
  dimension "d14" = 40
  dimension "d15" = 19
  dimension "d16" = 3.1
  dimension "d17" = 3.25
  dimension "d18" = 4
  dimension "d19" = 4
  dimension "d20" = 3.25
  dimension "d21" = 4
  dimension "d22" = 4
  dimension "d25" = 5.5
  constraint horizontal L4
  constraint vertical L5
  constraint horizontal L6
  constraint vertical L7
  constraint horizontal L8
  constraint vertical L9
  constraint horizontal L10
  constraint vertical L11
  constraint collinear L5 L9
  constraint collinear L7 L11
  constraint collinear L2 L6
  constraint collinear L0 L8
  constraint equal L5 L9
  constraint equal A0 A1
  constraint coincident A0.centre L12.start
  constraint coincident A1.centre L12.end
  constraint horizontal L12
  constraint equal A2 A3
  constraint equal A0 A2
  constraint coincident A2.centre L13.start
  constraint coincident A3.centre L13.end
  constraint parallel L4 L13
  constraint concentric A1 A5
  constraint equal A4 A5
  constraint equal A4 A6
  constraint equal A4 A7
  measures "d13" distance of L4.end L5.end
  measures "d14" distance of L9.end L10.end
  measures "d15" distance of L5 origin
  measures "d16" diameter of A0
  measures "d17" distance of L10 L12
  measures "d18" distance of L11 A0.centre
  measures "d19" distance of L9 A1.centre
  measures "d20" distance of L4 L13
  measures "d21" distance of L7 A2.centre
  measures "d22" distance of L5 A3.centre
  measures "d25" diameter of A4
extrude "Extrude3" add sketch "wing supports" against normal blind 3 separate body contours L0 L8 L9 L10 L11 | L2 L4 L5 L6 L7 | A4 | A5 | A6 | A7 makes body 2 at (18.1833, 22, -21) makes body 3 at (18.1833, 22, 21)
extrude "Extrude4" [suppressed]
equation "d5 = d4"
equation "d7 = margin"
equation "d8 = margin"
equation "d19 = d18"
equation "d20 = d17"
equation "d21 = d18"
equation "d22 = d18"

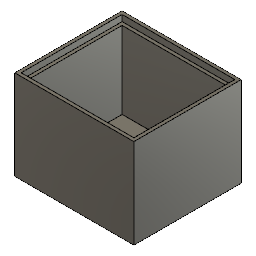
design "cover v2"
Autodesk Fusion 360 part; units mm, degrees
sketch "base" plane through (0, 0, 0) normal (0, 1, 0) x (1, 0, 0)
  line L0 (36.5, -32.9) -> (-36.5, -32.9)
  line L1 (-36.5, -32.9) -> (-36.5, -30.9)
  line L2 (-36.5, -30.9) -> (36.5, -30.9)
  line L3 (36.5, -30.9) -> (36.5, -32.9)
  line L4 (36.5, 32.9) -> (-36.5, 32.9)
  line L5 (-36.5, 32.9) -> (-36.5, 30.9)
  line L6 (-36.5, 30.9) -> (36.5, 30.9)
  line L7 (36.5, 30.9) -> (36.5, 32.9)
  line L8 (36.5, -30.9) -> (34.5, -30.9)
  line L9 (34.5, -30.9) -> (34.5, 30.9)
  line L10 (34.5, 30.9) -> (36.5, 30.9)
  line L11 (36.5, 30.9) -> (36.5, -30.9)
  line L12 (0, -49.6148) -> (0, 45.2004) construction
  line L13 (54.9351, 0) -> (-34.717, 0) construction
  line L14 (-36.5, -30.9) -> (-34.5, -30.9)
  line L15 (-34.5, -30.9) -> (-34.5, 30.9)
  line L16 (-34.5, 30.9) -> (-36.5, 30.9)
  line L17 (-36.5, 30.9) -> (-36.5, -30.9)
  dimension "d1" = 2
  dimension "d2" = 73
  dimension "d3" = 65.8
  constraint horizontal L0
  constraint vertical L1
  constraint horizontal L2
  constraint vertical L3
  constraint horizontal L4
  constraint vertical L5
  constraint horizontal L6
  constraint vertical L7
  constraint equal L3 L7
  constraint equal L2 L6
  constraint collinear L3 L7
  constraint horizontal L8
  constraint vertical L9
  constraint horizontal L10
  constraint vertical L11
  constraint coincident L6 L9.end
  constraint equal L3 L8
  constraint vertical L12
  constraint horizontal L13
  constraint coincident origin L13
  constraint coincident origin L12
  constraint symmetric L2 L6 L13
  constraint symmetric L1 L3 L12
  constraint horizontal L14
  constraint vertical L15
  constraint horizontal L16
  constraint vertical L17
  constraint coincident L6 L15.end
  constraint equal L8 L14
  measures "d1" distance of L0.start L2.end
  measures "d2" distance of L0.start L0.end
  measures "d3" distance of L0 L4
extrude "Extrude1" add sketch "base" along normal blind 55 contours L0 L1 L2 L3 L8 L14 | L2 L6 L8 L9 L10 L11 | L2 L6 L14 L15 L16 L17 | L4 L5 L6 L7 L10 L16 makes body 1
extrude "Extrude2" add sketch "base" along normal blind 4 separate body contours L2 L6 L9 L15 makes body 2
sketch "Sketch3" plane through (0, 4, 0) normal (0, 1, 0) x (-1, 0, 0)
  line L0 (-34.5, 30.9) -> (-34.5, -30.9)
  line L1 (-34.5, -30.9) -> (34.5, -30.9)
  line L2 (34.5, -30.9) -> (34.5, 30.9)
  line L3 (34.5, 30.9) -> (-34.5, 30.9)
  line L4 (-32.5, -28.9) -> (32.5, -28.9)
  line L5 (32.5, -28.9) -> (32.5, 28.9)
  line L6 (32.5, 28.9) -> (-32.5, 28.9)
  line L7 (-32.5, 28.9) -> (-32.5, -28.9)
  dimension "d16" = -2
extrude "Extrude5" add sketch "Sketch3" along normal blind 47.2 bodies 1 2
equation "d17 = 56 mm - 3.8 mm - 5 mm"
equation "d19 = 7.2 mm"
equation "d20 = d19"
equation "d21 = 14.15 mm - 0.2 mm"
equation "d22 = d21"

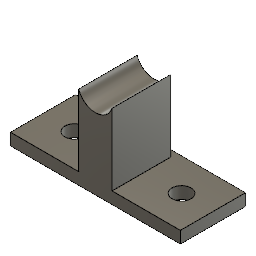
design "led cover"
Autodesk Fusion 360 part; units mm, degrees
sketch "Sketch1" plane through (0, 0, 0) normal (0, 1, 0) x (1, 0, 0)
  line L0 (2.5, -4.375) -> (-2.5, -4.375)
  line L1 (-2.5, -4.375) -> (-2.5, 4.375)
  line L2 (-2.5, 4.375) -> (2.5, 4.375)
  line L3 (2.5, 4.375) -> (2.5, -4.375)
  line L4 (0, -17.6215) -> (0, 10.113) construction
  line L5 (14.6118, 0) -> (-14.9327, 0) construction
  dimension "d1" = 5
  dimension "d2" = 8.75
  constraint horizontal L0
  constraint vertical L1
  constraint horizontal L2
  constraint vertical L3
  constraint parallel L1 L4
  constraint perpendicular L3 L5
  constraint coincident origin L5
  constraint coincident origin L4
  constraint symmetric L1 L3 L4
  constraint symmetric L0 L2 L5
  measures "d1" distance of L0.start L0.end
  measures "d2" distance of L0.end L1.end
extrude "Extrude1" add sketch "Sketch1" along normal blind 8.875
sketch "Sketch2" plane through (0, 0, 4.375) normal (0, 0, 1) x (1, 0, 0)
  line L0 (-2.5, 0) -> (2.5, 0)
  line L1 (2.5, 0) -> (2.5, 8.875)
  line L2 (2.5, 8.875) -> (-2.5, 8.875)
  line L3 (-2.5, 8.875) -> (-2.5, 0)
  line L4 (-2.5, 8.875) -> (2.5, 8.875)
  line L5 (2.5, 8.875) -> (2.5, 11.5)
  line L6 (2.5, 11.5) -> (-2.5, 11.5)
  line L7 (-2.5, 11.5) -> (-2.5, 8.875)
  circle A0 centre (0, 11.5) radius 2.625
  line L8 (0, 0) -> (0, 8.875) construction
  dimension "d10" = 5.25
  constraint horizontal L4
  constraint vertical L5
  constraint horizontal L6
  constraint vertical L7
  constraint coincident L2.end L3.start
  constraint tangent L4 A0
  constraint coincident L8.start origin
  constraint midpoint L4 L8.end
  constraint perpendicular L4 L8
  constraint coincident A0.centre L8
  constraint coincident L6 A0.centre
  measures "d10" diameter of A0
extrude "Extrude3" add sketch "Sketch2" against normal blind 8.75 contours L2 L4 L7 A0 | L2 L4 L5 A0
sketch "Sketch3" plane through (0, 0, 0) normal (0, -1, 0) x (1, 0, 0)
  line L0 (-2.5, -4.375) -> (2.5, -4.375)
  line L1 (2.5, -4.375) -> (2.5, 4.375)
  line L2 (2.5, 4.375) -> (-2.5, 4.375)
  line L3 (-2.5, 4.375) -> (-2.5, -4.375)
  line L4 (-12.7, 4.375) -> (12.7, 4.375)
  line L5 (12.7, 4.375) -> (12.7, -5.375)
  line L6 (12.7, -5.375) -> (-12.7, -5.375)
  line L7 (-12.7, -5.375) -> (-12.7, 4.375)
  line L8 (0, 4.375) -> (0, -4.375) construction
  line L9 (12.7, -0.5) -> (-12.7, -0.5) construction
  circle A0 centre (-8, -0.5) radius 1.42
  circle A1 centre (8, -0.5) radius 1.42
  dimension "d16" = 25.4
  dimension "d17" = 2.84
  dimension "d18" = 16
  dimension "d21" = 9.75
  dimension "d22" = 4.875
  constraint horizontal L4
  constraint vertical L5
  constraint horizontal L6
  constraint vertical L7
  constraint midpoint L2 L8.start
  constraint midpoint L0 L8.end
  constraint midpoint L4 L8.start
  constraint coincident L9 A0.centre
  constraint coincident L9 A1.centre
  constraint equal A0 A1
  constraint symmetric L8 A0 A1
  measures "d16" distance of L4.start L4.end
  measures "d17" diameter of A0
  measures "d18" distance of A0.centre A1.centre
  measures "d21" distance of L4.start L6.end
  measures "d22" distance of L4 L9
extrude "Extrude5" add sketch "Sketch3" along normal blind 1.8

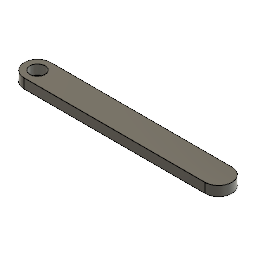
design "magnet storage latch"
Autodesk Fusion 360 part; units mm, degrees
sketch "Sketch1" plane through (0, 0, 0) normal (0, 1, 0) x (1, 0, 0)
  circle A0 centre (0, 0) radius 1.55
  circle A1 centre (0, 0) radius 2.75
  line L0 (0, 2.75) -> (37, 2.75)
  line L1 (29.0028, 0) -> (29.0028, 0)
  line L2 (37, -2.75) -> (0, -2.75)
  arc A2 (39.75, 0) -> (37, 2.75) centre (37, 0) ccw
  arc A3 (37, -2.75) -> (39.75, 0) centre (37, 0) ccw
  dimension "d1" = 3.1
  dimension "d3" = 5.5
  dimension "d4" = 2.75
  dimension "d6" = 37
  constraint coincident A0.centre A1.centre
  constraint concentric A0 A1
  constraint coincident A1 L0.start
  constraint horizontal L0
  constraint coincident A1 L2.end
  constraint tangent A1 L2
  constraint tangent A1 L0
  constraint horizontal L2
  constraint tangent L0 A2
  constraint tangent L2 A3
  constraint equal A2 A3
  constraint tangent A2 A3
  measures "d1" diameter of A0
  measures "d3" diameter of A1
  measures "d4" radius of A2
  measures "d6" distance of A0.centre A2.centre
extrude "Extrude1" add sketch "Sketch1" along normal blind 2
equation "d6 = 40 mm - d4 - 0.25 mm"
